Autodesk Fusion 360 part; units mm, degrees
note: some values were not read from the file. Chosen so that the rebuilt part matches the saved one: which bodies a step acts on.
(part 3 of 4)
sketch "BBB_22mm_Gearmotor_L_Section" plane through (0, 0, 0) normal (1, 0, 0) x (0, 0, -1) in component "BBB_22mm_Gearmotor_L"
  circle A0 centre (-21, 0) radius 11
extrude "Extrude1'''''''''''''''''''''''''''''''''''''''''''''''''''''''''''''''''''''" add sketch "BBB_22mm_Gearmotor_L_Section" along normal blind 49 from surface at -58 separate body makes body 78 in component "BBB_22mm_Gearmotor_L"
sketch "BBB_4mm_Output_Shaft_L_Section" plane through (0, 0, 0) normal (1, 0, 0) x (0, 0, -1) in component "BBB_4mm_Output_Shaft_L"
  circle A0 centre (-21, 0) radius 2
extrude "Extrude1''''''''''''''''''''''''''''''''''''''''''''''''''''''''''''''''''''''" add sketch "BBB_4mm_Output_Shaft_L_Section" along normal blind 14 from surface at -72 separate body makes body 79 in component "BBB_4mm_Output_Shaft_L"
sketch "BBB_Face_Mount_26mm_L_Outline" plane through (0, 0, 0) normal (0, 0, 1) x (1, 0, 0) in component "BBB_Face_Mount_26mm_L"
  line L0 (-61, -13) -> (-58, -13)
  line L1 (-58, -13) -> (-58, 13)
  line L2 (-58, 13) -> (-61, 13)
  line L3 (-61, 13) -> (-61, -13)
extrude "Extrude1'''''''''''''''''''''''''''''''''''''''''''''''''''''''''''''''''''''''" add sketch "BBB_Face_Mount_26mm_L_Outline" along normal blind 26 from surface at 8 separate body makes body 80 in component "BBB_Face_Mount_26mm_L"
sketch "Face_Motor_Bore_L" plane through (0, 0, 0) normal (1, 0, 0) x (0, 0, -1) in component "BBB_Face_Mount_26mm_L"
  circle A0 centre (-21, 0) radius 11.1
extrude "Face_Motor_Bore_L_Cut" cut sketch "Face_Motor_Bore_L" along normal blind 3.2 from surface at -61.1 bodies 80 in component "BBB_Face_Mount_26mm_L"
sketch "Face_M3_20mm_Pattern_L" plane through (0, 0, 0) normal (1, 0, 0) x (0, 0, -1) in component "BBB_Face_Mount_26mm_L"
  circle A0 centre (-11, -10) radius 1.6
  circle A1 centre (-31, -10) radius 1.6
  circle A2 centre (-11, 10) radius 1.6
  circle A3 centre (-31, 10) radius 1.6
extrude "Face_M3_20mm_Pattern_L_Cut" cut sketch "Face_M3_20mm_Pattern_L" along normal blind 3.2 from surface at -61.1 bodies 80 in component "BBB_Face_Mount_26mm_L"
sketch "BBB_Motor_Cradle_L_Outline" plane through (0, 0, 0) normal (0, 0, 1) x (1, 0, 0) in component "BBB_Motor_Cradle_L"
  line L0 (-58, -20) -> (-48, -20)
  line L1 (-48, -20) -> (-48, 20)
  line L2 (-48, 20) -> (-58, 20)
  line L3 (-58, 20) -> (-58, -20)
extrude "Extrude1''''''''''''''''''''''''''''''''''''''''''''''''''''''''''''''''''''''''" add sketch "BBB_Motor_Cradle_L_Outline" along normal blind 32 from surface at 5 separate body makes body 81 in component "BBB_Motor_Cradle_L"
sketch "Cradle_Motor_Bore_L" plane through (0, 0, 0) normal (1, 0, 0) x (0, 0, -1) in component "BBB_Motor_Cradle_L"
  circle A0 centre (-21, 0) radius 11.1
extrude "Cradle_Motor_Bore_L_Cut" cut sketch "Cradle_Motor_Bore_L" along normal blind 10.2 from surface at -58.1 bodies 81 in component "BBB_Motor_Cradle_L"
sketch "Cradle_M3_Face_Tap_L" plane through (0, 0, 0) normal (1, 0, 0) x (0, 0, -1) in component "BBB_Motor_Cradle_L"
  circle A0 centre (-11, -10) radius 1.25
  circle A1 centre (-31, -10) radius 1.25
  circle A2 centre (-11, 10) radius 1.25
  circle A3 centre (-31, 10) radius 1.25
extrude "Cradle_M3_Face_Tap_L_Cut" cut sketch "Cradle_M3_Face_Tap_L" along normal blind 10.2 from surface at -58.1 bodies 81 in component "BBB_Motor_Cradle_L"
sketch "Cradle_M3_Base_Tap_L" plane through (0, 0, 0) normal (0, 0, 1) x (1, 0, 0) in component "BBB_Motor_Cradle_L"
  circle A0 centre (-53, -16) radius 1.25
  circle A1 centre (-53, 16) radius 1.25
extrude "Cradle_M3_Base_Tap_L_Cut" cut sketch "Cradle_M3_Base_Tap_L" along normal blind 12.1 from surface at 4.9 bodies 81 in component "BBB_Motor_Cradle_L"
sketch "Cradle_M3_Base_Clear_L" plane through (0, 0, 0) normal (0, 0, 1) x (1, 0, 0) in component "Base_Plate_Al"
  circle A0 centre (-53, -16) radius 1.7
  circle A1 centre (-53, 16) radius 1.7
extrude "Cradle_M3_Base_Clear_L_Cut" cut sketch "Cradle_M3_Base_Clear_L" along normal blind 2.2 from surface at 2.9 bodies 1 in component "Base_Plate_Al"
sketch "Hub_16p2_Counterbore_L" plane through (0, 0, 0) normal (1, 0, 0) x (0, 0, -1) in component "Left_Wheel"
  circle A0 centre (-21, 0) radius 8.1
extrude "Hub_16p2_Counterbore_L_Cut" cut sketch "Hub_16p2_Counterbore_L" along normal blind 6.4 from surface at -67.2 bodies 4 in component "Left_Wheel"
sketch "Shaft_4p2_Blind_Bore_L" plane through (0, 0, 0) normal (1, 0, 0) x (0, 0, -1) in component "Left_Wheel"
  circle A0 centre (-21, 0) radius 2.1
extrude "Shaft_4p2_Blind_Bore_L_Cut" cut sketch "Shaft_4p2_Blind_Bore_L" along normal blind 5.1 from surface at -72.2 bodies 4 in component "Left_Wheel"
sketch "Wheel_M3_12p7_Pattern_L" plane through (0, 0, 0) normal (1, 0, 0) x (0, 0, -1) in component "Left_Wheel"
  circle A0 centre (-21, -6.35) radius 1.7
  circle A1 centre (-21, 6.35) radius 1.7
extrude "Wheel_M3_12p7_Pattern_L_Cut" cut sketch "Wheel_M3_12p7_Pattern_L" along normal blind 13 from surface at -80.1 bodies 4 in component "Left_Wheel"
sketch "Repeat_4mm_Clamp_Hub_L_Section" plane through (0, 0, 0) normal (1, 0, 0) x (0, 0, -1) in component "Repeat_4mm_Clamp_Hub_L"
  circle A0 centre (-21, 0) radius 8
extrude "Extrude1'''''''''''''''''''''''''''''''''''''''''''''''''''''''''''''''''''''''''" add sketch "Repeat_4mm_Clamp_Hub_L_Section" along normal blind 6 from surface at -67 separate body makes body 82 in component "Repeat_4mm_Clamp_Hub_L"
sketch "Hub_4mm_Shaft_Bore_L" plane through (0, 0, 0) normal (1, 0, 0) x (0, 0, -1) in component "Repeat_4mm_Clamp_Hub_L"
  circle A0 centre (-21, 0) radius 2
extrude "Hub_4mm_Shaft_Bore_L_Cut" cut sketch "Hub_4mm_Shaft_Bore_L" along normal blind 6.2 from surface at -67.1 bodies 82 in component "Repeat_4mm_Clamp_Hub_L"
sketch "Hub_M3_12p7_Tap_L" plane through (0, 0, 0) normal (1, 0, 0) x (0, 0, -1) in component "Repeat_4mm_Clamp_Hub_L"
  circle A0 centre (-21, -6.35) radius 1.25
  circle A1 centre (-21, 6.35) radius 1.25
extrude "Hub_M3_12p7_Tap_L_Cut" cut sketch "Hub_M3_12p7_Tap_L" along normal blind 6.2 from surface at -67.1 bodies 82 in component "Repeat_4mm_Clamp_Hub_L"
sketch "BBB_22mm_Gearmotor_R_Section" plane through (0, 0, 0) normal (1, 0, 0) x (0, 0, -1) in component "BBB_22mm_Gearmotor_R"
  circle A0 centre (-21, 0) radius 11
extrude "Extrude1''''''''''''''''''''''''''''''''''''''''''''''''''''''''''''''''''''''''''" add sketch "BBB_22mm_Gearmotor_R_Section" along normal blind 49 from surface at 9 separate body makes body 83 in component "BBB_22mm_Gearmotor_R"
sketch "BBB_4mm_Output_Shaft_R_Section" plane through (0, 0, 0) normal (1, 0, 0) x (0, 0, -1) in component "BBB_4mm_Output_Shaft_R"
  circle A0 centre (-21, 0) radius 2
extrude "Extrude1'''''''''''''''''''''''''''''''''''''''''''''''''''''''''''''''''''''''''''" add sketch "BBB_4mm_Output_Shaft_R_Section" along normal blind 14 from surface at 58 separate body makes body 84 in component "BBB_4mm_Output_Shaft_R"
sketch "BBB_Face_Mount_26mm_R_Outline" plane through (0, 0, 0) normal (0, 0, 1) x (1, 0, 0) in component "BBB_Face_Mount_26mm_R"
  line L0 (58, -13) -> (61, -13)
  line L1 (61, -13) -> (61, 13)
  line L2 (61, 13) -> (58, 13)
  line L3 (58, 13) -> (58, -13)
extrude "Extrude1''''''''''''''''''''''''''''''''''''''''''''''''''''''''''''''''''''''''''''" add sketch "BBB_Face_Mount_26mm_R_Outline" along normal blind 26 from surface at 8 separate body makes body 85 in component "BBB_Face_Mount_26mm_R"
sketch "Face_Motor_Bore_R" plane through (0, 0, 0) normal (1, 0, 0) x (0, 0, -1) in component "BBB_Face_Mount_26mm_R"
  circle A0 centre (-21, 0) radius 11.1
extrude "Face_Motor_Bore_R_Cut" cut sketch "Face_Motor_Bore_R" along normal blind 3.2 from surface at 57.9 bodies 85 in component "BBB_Face_Mount_26mm_R"
sketch "Face_M3_20mm_Pattern_R" plane through (0, 0, 0) normal (1, 0, 0) x (0, 0, -1) in component "BBB_Face_Mount_26mm_R"
  circle A0 centre (-11, -10) radius 1.6
  circle A1 centre (-31, -10) radius 1.6
  circle A2 centre (-11, 10) radius 1.6
  circle A3 centre (-31, 10) radius 1.6
extrude "Face_M3_20mm_Pattern_R_Cut" cut sketch "Face_M3_20mm_Pattern_R" along normal blind 3.2 from surface at 57.9 bodies 85 in component "BBB_Face_Mount_26mm_R"
sketch "BBB_Motor_Cradle_R_Outline" plane through (0, 0, 0) normal (0, 0, 1) x (1, 0, 0) in component "BBB_Motor_Cradle_R"
  line L0 (48, -20) -> (58, -20)
  line L1 (58, -20) -> (58, 20)
  line L2 (58, 20) -> (48, 20)
  line L3 (48, 20) -> (48, -20)
extrude "Extrude1'''''''''''''''''''''''''''''''''''''''''''''''''''''''''''''''''''''''''''''" add sketch "BBB_Motor_Cradle_R_Outline" along normal blind 32 from surface at 5 separate body makes body 86 in component "BBB_Motor_Cradle_R"
sketch "Cradle_Motor_Bore_R" plane through (0, 0, 0) normal (1, 0, 0) x (0, 0, -1) in component "BBB_Motor_Cradle_R"
  circle A0 centre (-21, 0) radius 11.1
extrude "Cradle_Motor_Bore_R_Cut" cut sketch "Cradle_Motor_Bore_R" along normal blind 10.2 from surface at 47.9 bodies 86 in component "BBB_Motor_Cradle_R"
sketch "Cradle_M3_Face_Tap_R" plane through (0, 0, 0) normal (1, 0, 0) x (0, 0, -1) in component "BBB_Motor_Cradle_R"
  circle A0 centre (-11, -10) radius 1.25
  circle A1 centre (-31, -10) radius 1.25
  circle A2 centre (-11, 10) radius 1.25
  circle A3 centre (-31, 10) radius 1.25
extrude "Cradle_M3_Face_Tap_R_Cut" cut sketch "Cradle_M3_Face_Tap_R" along normal blind 10.2 from surface at 47.9 bodies 86 in component "BBB_Motor_Cradle_R"
sketch "Cradle_M3_Base_Tap_R" plane through (0, 0, 0) normal (0, 0, 1) x (1, 0, 0) in component "BBB_Motor_Cradle_R"
  circle A0 centre (53, -16) radius 1.25
  circle A1 centre (53, 16) radius 1.25
extrude "Cradle_M3_Base_Tap_R_Cut" cut sketch "Cradle_M3_Base_Tap_R" along normal blind 12.1 from surface at 4.9 bodies 86 in component "BBB_Motor_Cradle_R"
sketch "Cradle_M3_Base_Clear_R" plane through (0, 0, 0) normal (0, 0, 1) x (1, 0, 0) in component "Base_Plate_Al"
  circle A0 centre (53, -16) radius 1.7
  circle A1 centre (53, 16) radius 1.7
extrude "Cradle_M3_Base_Clear_R_Cut" cut sketch "Cradle_M3_Base_Clear_R" along normal blind 2.2 from surface at 2.9 bodies 1 in component "Base_Plate_Al"
sketch "Hub_16p2_Counterbore_R" plane through (0, 0, 0) normal (1, 0, 0) x (0, 0, -1) in component "Right_Wheel"
  circle A0 centre (-21, 0) radius 8.1
extrude "Hub_16p2_Counterbore_R_Cut" cut sketch "Hub_16p2_Counterbore_R" along normal blind 6.4 from surface at 60.8 bodies 5 in component "Right_Wheel"
sketch "Shaft_4p2_Blind_Bore_R" plane through (0, 0, 0) normal (1, 0, 0) x (0, 0, -1) in component "Right_Wheel"
  circle A0 centre (-21, 0) radius 2.1
extrude "Shaft_4p2_Blind_Bore_R_Cut" cut sketch "Shaft_4p2_Blind_Bore_R" along normal blind 5.1 from surface at 67.1 bodies 5 in component "Right_Wheel"
sketch "Wheel_M3_12p7_Pattern_R" plane through (0, 0, 0) normal (1, 0, 0) x (0, 0, -1) in component "Right_Wheel"
  circle A0 centre (-21, -6.35) radius 1.7
  circle A1 centre (-21, 6.35) radius 1.7
extrude "Wheel_M3_12p7_Pattern_R_Cut" cut sketch "Wheel_M3_12p7_Pattern_R" along normal blind 13 from surface at 67.1 bodies 5 in component "Right_Wheel"
sketch "Repeat_4mm_Clamp_Hub_R_Section" plane through (0, 0, 0) normal (1, 0, 0) x (0, 0, -1) in component "Repeat_4mm_Clamp_Hub_R"
  circle A0 centre (-21, 0) radius 8
extrude "Extrude1''''''''''''''''''''''''''''''''''''''''''''''''''''''''''''''''''''''''''''''" add sketch "Repeat_4mm_Clamp_Hub_R_Section" along normal blind 6 from surface at 61 separate body makes body 87 in component "Repeat_4mm_Clamp_Hub_R"
sketch "Hub_4mm_Shaft_Bore_R" plane through (0, 0, 0) normal (1, 0, 0) x (0, 0, -1) in component "Repeat_4mm_Clamp_Hub_R"
  circle A0 centre (-21, 0) radius 2
extrude "Hub_4mm_Shaft_Bore_R_Cut" cut sketch "Hub_4mm_Shaft_Bore_R" along normal blind 6.2 from surface at 60.9 bodies 87 in component "Repeat_4mm_Clamp_Hub_R"
sketch "Hub_M3_12p7_Tap_R" plane through (0, 0, 0) normal (1, 0, 0) x (0, 0, -1) in component "Repeat_4mm_Clamp_Hub_R"
  circle A0 centre (-21, -6.35) radius 1.25
  circle A1 centre (-21, 6.35) radius 1.25
extrude "Hub_M3_12p7_Tap_R_Cut" cut sketch "Hub_M3_12p7_Tap_R" along normal blind 6.2 from surface at 60.9 bodies 87 in component "Repeat_4mm_Clamp_Hub_R"
sketch "BBB_Dual_Brushed_ESC_v2_Envelope_Outline" plane through (0, 0, 0) normal (0, 0, 1) x (1, 0, 0) in component "BBB_Dual_Brushed_ESC_v2_Envelope"
  line L0 (-8, -84) -> (12, -84)
  line L1 (12, -84) -> (12, -68)
  line L2 (12, -68) -> (-8, -68)
  line L3 (-8, -68) -> (-8, -84)
extrude "Extrude1'''''''''''''''''''''''''''''''''''''''''''''''''''''''''''''''''''''''''''''''" add sketch "BBB_Dual_Brushed_ESC_v2_Envelope_Outline" along normal blind 5 from surface at 7 separate body makes body 88 in component "BBB_Dual_Brushed_ESC_v2_Envelope"
sketch "Battery_Tray_Rear_Clearance_L" plane through (0, 0, 0) normal (0, 0, 1) x (1, 0, 0) in component "BBB_Motor_Cradle_L"
  line L0 (-58.1, -20.1) -> (-47.9, -20.1)
  line L1 (-47.9, -20.1) -> (-47.9, -18)
  line L2 (-47.9, -18) -> (-58.1, -18)
  line L3 (-58.1, -18) -> (-58.1, -20.1)
extrude "Extrude5''''''''''''''" cut sketch "Battery_Tray_Rear_Clearance_L" along normal blind 7.1 from surface at 30 bodies 81 in component "BBB_Motor_Cradle_L"
sketch "Battery_Tray_Rear_Clearance_R" plane through (0, 0, 0) normal (0, 0, 1) x (1, 0, 0) in component "BBB_Motor_Cradle_R"
  line L0 (47.9, -20.1) -> (58.1, -20.1)
  line L1 (58.1, -20.1) -> (58.1, -18)
  line L2 (58.1, -18) -> (47.9, -18)
  line L3 (47.9, -18) -> (47.9, -20.1)
extrude "Extrude5'''''''''''''''" cut sketch "Battery_Tray_Rear_Clearance_R" along normal blind 7.1 from surface at 30 bodies 86 in component "BBB_Motor_Cradle_R"
sketch "Battery_Clamp_Bar_1_Outline" plane through (0, 0, 0) normal (0, 0, 1) x (1, 0, 0) in component "Battery_Clamp_Bar_1"
  line L0 (-78, -51) -> (78, -51)
  line L1 (78, -51) -> (78, -45)
  line L2 (78, -45) -> (-78, -45)
  line L3 (-78, -45) -> (-78, -51)
extrude "Extrude1''''''''''''''''''''''''''''''''''''''''''''''''''''''''''''''''''''''''''''''''" add sketch "Battery_Clamp_Bar_1_Outline" along normal blind 6 from surface at 61.6 separate body makes body 89 in component "Battery_Clamp_Bar_1"
sketch "Clamp_M3_Tap_L_1" plane through (0, 0, 0) normal (1, 0, 0) x (0, 0, -1) in component "Battery_Clamp_Bar_1"
  circle A0 centre (-64.6, -48) radius 1.25
extrude "Extrude2'''''''''''''''''''''''''''''''''''''''''''''''''" cut sketch "Clamp_M3_Tap_L_1" along normal blind 10.2 from surface at -78.1 bodies 89 in component "Battery_Clamp_Bar_1"
sketch "Clamp_M3_Tap_R_1" plane through (0, 0, 0) normal (1, 0, 0) x (0, 0, -1) in component "Battery_Clamp_Bar_1"
  circle A0 centre (-64.6, -48) radius 1.25
extrude "Extrude3''''''''''''''''''''''''''''" cut sketch "Clamp_M3_Tap_R_1" along normal blind 10.2 from surface at 67.9 bodies 89 in component "Battery_Clamp_Bar_1"
sketch "Clamp_M3_Clear_L_1" plane through (0, 0, 0) normal (1, 0, 0) x (0, 0, -1) in component "Left_Side_Plate_Al"
  circle A0 centre (-64.6, -48) radius 1.7
extrude "Extrude8'''" cut sketch "Clamp_M3_Clear_L_1" along normal blind 2.2 from surface at -80.1 bodies 2 in component "Left_Side_Plate_Al"
sketch "Clamp_M3_Clear_R_1" plane through (0, 0, 0) normal (1, 0, 0) x (0, 0, -1) in component "Right_Side_Plate_Al"
  circle A0 centre (-64.6, -48) radius 1.7
extrude "Extrude8''''" cut sketch "Clamp_M3_Clear_R_1" along normal blind 2.2 from surface at 77.9 bodies 3 in component "Right_Side_Plate_Al"
sketch "Battery_Clamp_Bar_2_Outline" plane through (0, 0, 0) normal (0, 0, 1) x (1, 0, 0) in component "Battery_Clamp_Bar_2"
  line L0 (-78, -31) -> (78, -31)
  line L1 (78, -31) -> (78, -25)
  line L2 (78, -25) -> (-78, -25)
  line L3 (-78, -25) -> (-78, -31)
extrude "Extrude1'''''''''''''''''''''''''''''''''''''''''''''''''''''''''''''''''''''''''''''''''" add sketch "Battery_Clamp_Bar_2_Outline" along normal blind 6 from surface at 61.6 separate body makes body 90 in component "Battery_Clamp_Bar_2"
sketch "Clamp_M3_Tap_L_2" plane through (0, 0, 0) normal (1, 0, 0) x (0, 0, -1) in component "Battery_Clamp_Bar_2"
  circle A0 centre (-64.6, -28) radius 1.25
extrude "Extrude2''''''''''''''''''''''''''''''''''''''''''''''''''" cut sketch "Clamp_M3_Tap_L_2" along normal blind 10.2 from surface at -78.1 bodies 90 in component "Battery_Clamp_Bar_2"
sketch "Clamp_M3_Tap_R_2" plane through (0, 0, 0) normal (1, 0, 0) x (0, 0, -1) in component "Battery_Clamp_Bar_2"
  circle A0 centre (-64.6, -28) radius 1.25
extrude "Extrude3'''''''''''''''''''''''''''''" cut sketch "Clamp_M3_Tap_R_2" along normal blind 10.2 from surface at 67.9 bodies 90 in component "Battery_Clamp_Bar_2"
sketch "Clamp_M3_Clear_L_2" plane through (0, 0, 0) normal (1, 0, 0) x (0, 0, -1) in component "Left_Side_Plate_Al"
  circle A0 centre (-64.6, -28) radius 1.7
extrude "Extrude9'" cut sketch "Clamp_M3_Clear_L_2" along normal blind 2.2 from surface at -80.1 bodies 2 in component "Left_Side_Plate_Al"
sketch "Clamp_M3_Clear_R_2" plane through (0, 0, 0) normal (1, 0, 0) x (0, 0, -1) in component "Right_Side_Plate_Al"
  circle A0 centre (-64.6, -28) radius 1.7
extrude "Extrude9''" cut sketch "Clamp_M3_Clear_R_2" along normal blind 2.2 from surface at 77.9 bodies 3 in component "Right_Side_Plate_Al"
sketch "Lifter_Servo_Clamp_Bar_L_Outline" plane through (0, 0, 0) normal (0, 0, 1) x (1, 0, 0) in component "Lifter_Servo_Clamp_Bar_L"
  line L0 (-15, -15) -> (-9, -15)
  line L1 (-9, -15) -> (-9, 60)
  line L2 (-9, 60) -> (-15, 60)
  line L3 (-15, 60) -> (-15, -15)
extrude "Extrude1''''''''''''''''''''''''''''''''''''''''''''''''''''''''''''''''''''''''''''''''''" add sketch "Lifter_Servo_Clamp_Bar_L_Outline" along normal blind 2 from surface at 32 separate body makes body 91 in component "Lifter_Servo_Clamp_Bar_L"
sketch "Clamp_Bar_M3_Clear_L" plane through (0, 0, 0) normal (0, 0, 1) x (1, 0, 0) in component "Lifter_Servo_Clamp_Bar_L"
  circle A0 centre (-12, -15) radius 1.7
  circle A1 centre (-12, 60) radius 1.7
extrude "Extrude2'''''''''''''''''''''''''''''''''''''''''''''''''''" cut sketch "Clamp_Bar_M3_Clear_L" along normal blind 2.2 from surface at 31.9 bodies 91 in component "Lifter_Servo_Clamp_Bar_L"
sketch "Lifter_Servo_Clamp_Post_L_Rear_Outline" plane through (0, 0, 0) normal (0, 0, 1) x (1, 0, 0) in component "Lifter_Servo_Clamp_Post_L_Rear"
  line L0 (-15, -18) -> (-9, -18)
  line L1 (-9, -18) -> (-9, -12)
  line L2 (-9, -12) -> (-15, -12)
  line L3 (-15, -12) -> (-15, -18)
extrude "Extrude1'''''''''''''''''''''''''''''''''''''''''''''''''''''''''''''''''''''''''''''''''''" add sketch "Lifter_Servo_Clamp_Post_L_Rear_Outline" along normal blind 27 from surface at 5 separate body makes body 92 in component "Lifter_Servo_Clamp_Post_L_Rear"
sketch "Clamp_Post_M3_Tap_L_Rear" plane through (0, 0, 0) normal (0, 0, 1) x (1, 0, 0) in component "Lifter_Servo_Clamp_Post_L_Rear"
  circle A0 centre (-12, -15) radius 1.25
extrude "Extrude2''''''''''''''''''''''''''''''''''''''''''''''''''''" cut sketch "Clamp_Post_M3_Tap_L_Rear" along normal blind 27.2 from surface at 4.9 bodies 92 in component "Lifter_Servo_Clamp_Post_L_Rear"
sketch "Lifter_Servo_Clamp_Post_L_Front_Outline" plane through (0, 0, 0) normal (0, 0, 1) x (1, 0, 0) in component "Lifter_Servo_Clamp_Post_L_Front"
  line L0 (-15, 57) -> (-9, 57)
  line L1 (-9, 57) -> (-9, 63)
  line L2 (-9, 63) -> (-15, 63)
  line L3 (-15, 63) -> (-15, 57)
extrude "Extrude1''''''''''''''''''''''''''''''''''''''''''''''''''''''''''''''''''''''''''''''''''''" add sketch "Lifter_Servo_Clamp_Post_L_Front_Outline" along normal blind 27 from surface at 5 separate body makes body 93 in component "Lifter_Servo_Clamp_Post_L_Front"
sketch "Clamp_Post_M3_Tap_L_Front" plane through (0, 0, 0) normal (0, 0, 1) x (1, 0, 0) in component "Lifter_Servo_Clamp_Post_L_Front"
  circle A0 centre (-12, 60) radius 1.25
extrude "Extrude2'''''''''''''''''''''''''''''''''''''''''''''''''''''" cut sketch "Clamp_Post_M3_Tap_L_Front" along normal blind 27.2 from surface at 4.9 bodies 93 in component "Lifter_Servo_Clamp_Post_L_Front"
sketch "Lifter_Servo_Clamp_Bar_R_Outline" plane through (0, 0, 0) normal (0, 0, 1) x (1, 0, 0) in component "Lifter_Servo_Clamp_Bar_R"
  line L0 (9, -15) -> (15, -15)
  line L1 (15, -15) -> (15, 60)
  line L2 (15, 60) -> (9, 60)
  line L3 (9, 60) -> (9, -15)
extrude "Extrude1'''''''''''''''''''''''''''''''''''''''''''''''''''''''''''''''''''''''''''''''''''''" add sketch "Lifter_Servo_Clamp_Bar_R_Outline" along normal blind 2 from surface at 32 separate body makes body 94 in component "Lifter_Servo_Clamp_Bar_R"
sketch "Clamp_Bar_M3_Clear_R" plane through (0, 0, 0) normal (0, 0, 1) x (1, 0, 0) in component "Lifter_Servo_Clamp_Bar_R"
  circle A0 centre (12, -15) radius 1.7
  circle A1 centre (12, 60) radius 1.7
extrude "Extrude2''''''''''''''''''''''''''''''''''''''''''''''''''''''" cut sketch "Clamp_Bar_M3_Clear_R" along normal blind 2.2 from surface at 31.9 bodies 94 in component "Lifter_Servo_Clamp_Bar_R"
sketch "Lifter_Servo_Clamp_Post_R_Rear_Outline" plane through (0, 0, 0) normal (0, 0, 1) x (1, 0, 0) in component "Lifter_Servo_Clamp_Post_R_Rear"
  line L0 (9, -18) -> (15, -18)
  line L1 (15, -18) -> (15, -12)
  line L2 (15, -12) -> (9, -12)
  line L3 (9, -12) -> (9, -18)
extrude "Extrude1''''''''''''''''''''''''''''''''''''''''''''''''''''''''''''''''''''''''''''''''''''''" add sketch "Lifter_Servo_Clamp_Post_R_Rear_Outline" along normal blind 27 from surface at 5 separate body makes body 95 in component "Lifter_Servo_Clamp_Post_R_Rear"
sketch "Clamp_Post_M3_Tap_R_Rear" plane through (0, 0, 0) normal (0, 0, 1) x (1, 0, 0) in component "Lifter_Servo_Clamp_Post_R_Rear"
  circle A0 centre (12, -15) radius 1.25
extrude "Extrude2'''''''''''''''''''''''''''''''''''''''''''''''''''''''" cut sketch "Clamp_Post_M3_Tap_R_Rear" along normal blind 27.2 from surface at 4.9 bodies 95 in component "Lifter_Servo_Clamp_Post_R_Rear"
sketch "Lifter_Servo_Clamp_Post_R_Front_Outline" plane through (0, 0, 0) normal (0, 0, 1) x (1, 0, 0) in component "Lifter_Servo_Clamp_Post_R_Front"
  line L0 (9, 57) -> (15, 57)
  line L1 (15, 57) -> (15, 63)
  line L2 (15, 63) -> (9, 63)
  line L3 (9, 63) -> (9, 57)
extrude "Extrude1'''''''''''''''''''''''''''''''''''''''''''''''''''''''''''''''''''''''''''''''''''''''" add sketch "Lifter_Servo_Clamp_Post_R_Front_Outline" along normal blind 27 from surface at 5 separate body makes body 96 in component "Lifter_Servo_Clamp_Post_R_Front"
sketch "Clamp_Post_M3_Tap_R_Front" plane through (0, 0, 0) normal (0, 0, 1) x (1, 0, 0) in component "Lifter_Servo_Clamp_Post_R_Front"
  circle A0 centre (12, 60) radius 1.25
extrude "Extrude2''''''''''''''''''''''''''''''''''''''''''''''''''''''''" cut sketch "Clamp_Post_M3_Tap_R_Front" along normal blind 27.2 from surface at 4.9 bodies 96 in component "Lifter_Servo_Clamp_Post_R_Front"
sketch "Lifter_Servo_Clamp_Base_M3_Clear" plane through (0, 0, 0) normal (0, 0, 1) x (1, 0, 0) in component "Base_Plate_Al"
  circle A0 centre (-12, -15) radius 1.7
  circle A1 centre (-12, 60) radius 1.7
  circle A2 centre (12, -15) radius 1.7
  circle A3 centre (12, 60) radius 1.7
extrude "Extrude33" cut sketch "Lifter_Servo_Clamp_Base_M3_Clear" along normal blind 2.2 from surface at 2.9 bodies 1 in component "Base_Plate_Al"
sketch "Pin_Clip_Groove_L" plane through (0, 0, 0) normal (1, 0, 0) x (0, 0, -1) in component "Lifter_Pivot_Pin_6mm"
  circle A0 centre (-31.5, 68) radius 3.05
  circle A1 centre (-31.5, 68) radius 2.5
extrude "Extrude4''''''''''''''''''''" cut sketch "Pin_Clip_Groove_L" along normal blind 0.8 from surface at -31.4 bodies 60 in component "Lifter_Pivot_Pin_6mm"
sketch "Pin_Clip_Groove_R" plane through (0, 0, 0) normal (1, 0, 0) x (0, 0, -1) in component "Lifter_Pivot_Pin_6mm"
  circle A0 centre (-31.5, 68) radius 3.05
  circle A1 centre (-31.5, 68) radius 2.5
extrude "Extrude5''''''''''''''''" cut sketch "Pin_Clip_Groove_R" along normal blind 0.8 from surface at 30.6 bodies 60 in component "Lifter_Pivot_Pin_6mm"
sketch "C_Clip_Section_L" plane through (0, 0, 0) normal (1, 0, 0) x (0, 0, -1) in component "Lifter_Pin_C_Clip_L"
  circle A0 centre (-31.5, 68) radius 5
  circle A1 centre (-31.5, 68) radius 2.5
extrude "Extrude1''''''''''''''''''''''''''''''''''''''''''''''''''''''''''''''''''''''''''''''''''''''''" add sketch "C_Clip_Section_L" along normal blind 0.8 from surface at -31.4 separate body makes body 97 in component "Lifter_Pin_C_Clip_L"
sketch "C_Clip_Opening_L" plane through (0, 0, 0) normal (1, 0, 0) x (0, 0, -1) in component "Lifter_Pin_C_Clip_L"
  line L0 (-30.4, 70.2) -> (-32.6, 70.2)
  line L1 (-32.6, 70.2) -> (-32.6, 73.2)
  line L2 (-32.6, 73.2) -> (-30.4, 73.2)
  line L3 (-30.4, 73.2) -> (-30.4, 70.2)
extrude "Extrude2'''''''''''''''''''''''''''''''''''''''''''''''''''''''''" cut sketch "C_Clip_Opening_L" along normal blind 1 from surface at -31.5 bodies 97 in component "Lifter_Pin_C_Clip_L"
sketch "C_Clip_Section_R" plane through (0, 0, 0) normal (1, 0, 0) x (0, 0, -1) in component "Lifter_Pin_C_Clip_R"
  circle A0 centre (-31.5, 68) radius 5
  circle A1 centre (-31.5, 68) radius 2.5
extrude "Extrude1'''''''''''''''''''''''''''''''''''''''''''''''''''''''''''''''''''''''''''''''''''''''''" add sketch "C_Clip_Section_R" along normal blind 0.8 from surface at 30.6 separate body makes body 98 in component "Lifter_Pin_C_Clip_R"
sketch "C_Clip_Opening_R" plane through (0, 0, 0) normal (1, 0, 0) x (0, 0, -1) in component "Lifter_Pin_C_Clip_R"
  line L0 (-30.4, 70.2) -> (-32.6, 70.2)
  line L1 (-32.6, 70.2) -> (-32.6, 73.2)
  line L2 (-32.6, 73.2) -> (-30.4, 73.2)
  line L3 (-30.4, 73.2) -> (-30.4, 70.2)
extrude "Extrude2''''''''''''''''''''''''''''''''''''''''''''''''''''''''''" cut sketch "C_Clip_Opening_R" along normal blind 1 from surface at 30.5 bodies 98 in component "Lifter_Pin_C_Clip_R"
sketch "C_Clip_OD_8p4_L" plane through (0, 0, 0) normal (1, 0, 0) x (0, 0, -1) in component "Lifter_Pin_C_Clip_L"
  circle A0 centre (-31.5, 68) radius 5.1
  circle A1 centre (-31.5, 68) radius 4.2
extrude "Extrude3''''''''''''''''''''''''''''''" cut sketch "C_Clip_OD_8p4_L" along normal blind 1 from surface at -31.5 bodies 97 in component "Lifter_Pin_C_Clip_L"
sketch "C_Clip_OD_8p4_R" plane through (0, 0, 0) normal (1, 0, 0) x (0, 0, -1) in component "Lifter_Pin_C_Clip_R"
  circle A0 centre (-31.5, 68) radius 5.1
  circle A1 centre (-31.5, 68) radius 4.2
extrude "Extrude3'''''''''''''''''''''''''''''''" cut sketch "C_Clip_OD_8p4_R" along normal blind 1 from surface at 30.5 bodies 98 in component "Lifter_Pin_C_Clip_R"
sketch "C_Clip_OD_8p0_L" plane through (0, 0, 0) normal (1, 0, 0) x (0, 0, -1) in component "Lifter_Pin_C_Clip_L"
  circle A0 centre (-31.5, 68) radius 5.1
  circle A1 centre (-31.5, 68) radius 4
extrude "Extrude4'''''''''''''''''''''" cut sketch "C_Clip_OD_8p0_L" along normal blind 1 from surface at -31.5 bodies 97 in component "Lifter_Pin_C_Clip_L"
sketch "C_Clip_OD_8p0_R" plane through (0, 0, 0) normal (1, 0, 0) x (0, 0, -1) in component "Lifter_Pin_C_Clip_R"
  circle A0 centre (-31.5, 68) radius 5.1
  circle A1 centre (-31.5, 68) radius 4
extrude "Extrude4''''''''''''''''''''''" cut sketch "C_Clip_OD_8p0_R" along normal blind 1 from surface at 30.5 bodies 98 in component "Lifter_Pin_C_Clip_R"
component "01_Chassis" placed x (1, 0, 0) y (0, 1, 0) z (0, 0, 1) at (0, 0, 0)
component "02_Drivetrain" placed x (1, 0, 0) y (0, 1, 0) z (0, 0, 1) at (0, 0, 0)
component "03_Front_Spinner" placed x (1, 0, 0) y (0, 1, 0) z (0, 0, 1) at (0, 0, 0)
component "05_Electronics" placed x (1, 0, 0) y (0, 1, 0) z (0, 0, 1) at (0, 0, 0)
component "06_3D_Printed" placed x (1, 0, 0) y (0, 1, 0) z (0, 0, 1) at (0, 0, 0)
component "07_Wedge_Lifter_Option" placed x (1, 0, 0) y (0, 1, 0) z (0, 0, 1) at (0, 0, 0)
component "08_Grabber_Addon_Option" placed x (1, 0, 0) y (0, 1, 0) z (0, 0, 1) at (0, 0, 0)
component "09_3S_Drive_Upgrade" placed x (1, 0, 0) y (0, 1, 0) z (0, 0, 1) at (0, 0, 0)
component "10_Battery_Restraints" placed x (1, 0, 0) y (0, 1, 0) z (0, 0, 1) at (0, 0, 0)
component "Base_Plate_Al" placed x (1, 0, 0) y (0, 1, 0) z (0, 0, 1) at (0, 0, 0) in component "01_Chassis"
component "Left_Side_Plate_Al" placed x (1, 0, 0) y (0, 1, 0) z (0, 0, 1) at (0, 0, 0) in component "01_Chassis"
component "Right_Side_Plate_Al" placed x (1, 0, 0) y (0, 1, 0) z (0, 0, 1) at (0, 0, 0) in component "01_Chassis"
component "Top_Cover" placed x (1, 0, 0) y (0, 1, 0) z (0, 0, 1) at (0, 0, 0) in component "01_Chassis"
component "Front_Wedge_L" placed x (1, 0, 0) y (0, 1, 0) z (0, 0, 1) at (0, 0, 0) in component "01_Chassis"
component "Front_Wedge_R" placed x (1, 0, 0) y (0, 1, 0) z (0, 0, 1) at (0, 0, 0) in component "01_Chassis"
component "Standoffs_Fasteners" placed x (1, 0, 0) y (0, 1, 0) z (0, 0, 1) at (0, 0, 0) in component "01_Chassis"
component "Left_Wheel" placed x (1, 0, 0) y (0, 1, 0) z (0, 0, 1) at (0, 0, 0) in component "02_Drivetrain"
component "Right_Wheel" placed x (1, 0, 0) y (0, 1, 0) z (0, 0, 1) at (0, 0, 0) in component "02_Drivetrain"
component "TT_Gearbox_L" placed x (1, 0, 0) y (0, 1, 0) z (0, 0, 1) at (0, 0, 0) in component "02_Drivetrain"
component "TT_Motor_Can_L" placed x (1, 0, 0) y (0, 1, 0) z (0, 0, 1) at (0, 0, 0) in component "02_Drivetrain"
component "TT_Gearbox_R" placed x (1, 0, 0) y (0, 1, 0) z (0, 0, 1) at (0, 0, 0) in component "02_Drivetrain"
component "TT_Motor_Can_R" placed x (1, 0, 0) y (0, 1, 0) z (0, 0, 1) at (0, 0, 0) in component "02_Drivetrain"
component "TT_Motor_Mount_L" placed x (1, 0, 0) y (0, 1, 0) z (0, 0, 1) at (0, 0, 0) in component "02_Drivetrain"
component "TT_Motor_Clamp_L" placed x (1, 0, 0) y (0, 1, 0) z (0, 0, 1) at (0, 0, 0) in component "02_Drivetrain"
component "TT_Motor_Mount_R" placed x (1, 0, 0) y (0, 1, 0) z (0, 0, 1) at (0, 0, 0) in component "02_Drivetrain"
component "TT_Motor_Clamp_R" placed x (1, 0, 0) y (0, 1, 0) z (0, 0, 1) at (0, 0, 0) in component "02_Drivetrain"
component "Spinner_Shaft" placed x (1, 0, 0) y (0, 1, 0) z (0, 0, 1) at (0, 0, 0) in component "03_Front_Spinner"
component "Left_Support" placed x (1, 0, 0) y (0, 1, 0) z (0, 0, 1) at (0, 0, 0) in component "03_Front_Spinner"
component "Right_Support" placed x (1, 0, 0) y (0, 1, 0) z (0, 0, 1) at (0, 0, 0) in component "03_Front_Spinner"
component "Spinner_Motor" placed x (1, 0, 0) y (0, 1, 0) z (0, 0, 1) at (0, 0, 0) in component "03_Front_Spinner"
component "Spinner_Motor_Cradle" placed x (1, 0, 0) y (0, 1, 0) z (0, 0, 1) at (0, 0, 0) in component "03_Front_Spinner"
component "Weapon_Pulley" placed x (1, 0, 0) y (0, 1, 0) z (0, 0, 1) at (0, 0, 0) in component "03_Front_Spinner"
component "Motor_Pulley" placed x (1, 0, 0) y (0, 1, 0) z (0, 0, 1) at (0, 0, 0) in component "03_Front_Spinner"
component "ESC_Tekko32" placed x (1, 0, 0) y (0, 1, 0) z (0, 0, 1) at (0, 0, 0) in component "03_Front_Spinner"
component "Spinner_Bar" placed x (1, 0, 0) y (0, 1, 0) z (0, 0, 1) at (0, 0, 0) in component "03_Front_Spinner"
component "Spinner_Sweep_Envelope" placed x (1, 0, 0) y (0, 1, 0) z (0, 0, 1) at (0, 0, 0) in component "03_Front_Spinner"
component "Cable_Routing_Keepouts" placed x (1, 0, 0) y (0, 1, 0) z (0, 0, 1) at (0, 0, 0) in component "05_Electronics"
component "Battery_and_Tray" placed x (1, 0, 0) y (0, 1, 0) z (0, 0, 1) at (0, 0, 0) in component "05_Electronics"
component "Rx_ER6" placed x (1, 0, 0) y (0, 1, 0) z (0, 0, 1) at (0, 0, 0) in component "05_Electronics"
component "UBEC_5A" placed x (1, 0, 0) y (0, 1, 0) z (0, 0, 1) at (0, 0, 0) in component "05_Electronics"
component "DRV8874_A" placed x (1, 0, 0) y (0, 1, 0) z (0, 0, 1) at (0, 0, 0) in component "05_Electronics"
component "DRV8874_B" placed x (1, 0, 0) y (0, 1, 0) z (0, 0, 1) at (0, 0, 0) in component "05_Electronics"
component "ESP32_DevKit" placed x (1, 0, 0) y (0, 1, 0) z (0, 0, 1) at (0, 0, 0) in component "05_Electronics"
component "FingerTech_Mini_Switch_Envelope" placed x (1, 0, 0) y (0, 1, 0) z (0, 0, 1) at (0, 0, 0) in component "05_Electronics"
component "BBB_Dual_Brushed_ESC_v2_Envelope" placed x (1, 0, 0) y (0, 1, 0) z (0, 0, 1) at (0, 0, 0) in component "05_Electronics"
component "Wire_Clips" placed x (1, 0, 0) y (0, 1, 0) z (0, 0, 1) at (0, 0, 0) in component "06_3D_Printed"
component "Non_Structural_Covers" placed x (1, 0, 0) y (0, 1, 0) z (0, 0, 1) at (0, 0, 0) in component "06_3D_Printed"
component "TPU_Bumpers" placed x (1, 0, 0) y (0, 1, 0) z (0, 0, 1) at (0, 0, 0) in component "06_3D_Printed"
component "Battery_Holder" placed x (1, 0, 0) y (0, 1, 0) z (0, 0, 1) at (0, 0, 0) in component "06_3D_Printed"
component "Batt_Post_1" placed x (1, 0, 0) y (0, 1, 0) z (0, 0, 1) at (0, 0, 0) in component "06_3D_Printed"
component "Batt_Post_2" placed x (1, 0, 0) y (0, 1, 0) z (0, 0, 1) at (0, 0, 0) in component "06_3D_Printed"
component "Batt_Post_3" placed x (1, 0, 0) y (0, 1, 0) z (0, 0, 1) at (0, 0, 0) in component "06_3D_Printed"
component "Batt_Post_4" placed x (1, 0, 0) y (0, 1, 0) z (0, 0, 1) at (0, 0, 0) in component "06_3D_Printed"
component "Disconnect_Post_1" placed x (1, 0, 0) y (0, 1, 0) z (0, 0, 1) at (0, 0, 0) in component "06_3D_Printed"
component "Disconnect_Post_2" placed x (1, 0, 0) y (0, 1, 0) z (0, 0, 1) at (0, 0, 0) in component "06_3D_Printed"
component "Holder_ESC_Tekko32" placed x (1, 0, 0) y (0, 1, 0) z (0, 0, 1) at (0, 0, 0) in component "06_3D_Printed"
component "Holder_Rx_ER6" placed x (1, 0, 0) y (0, 1, 0) z (0, 0, 1) at (0, 0, 0) in component "06_3D_Printed"
component "Holder_UBEC_5A" placed x (1, 0, 0) y (0, 1, 0) z (0, 0, 1) at (0, 0, 0) in component "06_3D_Printed"
component "Holder_DRV8874_A" placed x (1, 0, 0) y (0, 1, 0) z (0, 0, 1) at (0, 0, 0) in component "06_3D_Printed"
component "Holder_DRV8874_B" placed x (1, 0, 0) y (0, 1, 0) z (0, 0, 1) at (0, 0, 0) in component "06_3D_Printed"
component "Holder_ESP32" placed x (1, 0, 0) y (0, 1, 0) z (0, 0, 1) at (0, 0, 0) in component "06_3D_Printed"
component "FingerTech_Switch_Adapter" placed x (1, 0, 0) y (0, 1, 0) z (0, 0, 1) at (0, 0, 0) in component "06_3D_Printed"
component "Rear_Panel" placed x (1, 0, 0) y (0, 1, 0) z (0, 0, 1) at (0, 0, 0) in component "Non_Structural_Covers"
component "06_3D_Printed" placed x (1, 0, 0) y (0, 1, 0) z (0, 0, 1) at (0, 0, 0) in component "TPU_Bumpers"
component "Lifter_Spatula_62mm" placed x (1, 0, 0) y (0, 1, 0) z (0, 0, 1) at (0, 0, 0) in component "07_Wedge_Lifter_Option"
component "Lifter_Hinge_Boss" placed x (1, 0, 0) y (0, 1, 0) z (0, 0, 1) at (0, 0, 0) in component "07_Wedge_Lifter_Option"
component "Lifter_Pivot_Support_L" placed x (1, 0, 0) y (0, 1, 0) z (0, 0, 1) at (0, 0, 0) in component "07_Wedge_Lifter_Option"
component "Lifter_Pivot_Support_R" placed x (1, 0, 0) y (0, 1, 0) z (0, 0, 1) at (0, 0, 0) in component "07_Wedge_Lifter_Option"
component "Lifter_Pivot_Pin_6mm" placed x (1, 0, 0) y (0, 1, 0) z (0, 0, 1) at (0, 0, 0) in component "07_Wedge_Lifter_Option"
component "Servo_30kgcm_Envelope_Only" placed x (1, 0, 0) y (0, 1, 0) z (0, 0, 1) at (0, 0, 0) in component "07_Wedge_Lifter_Option"
component "Lifter_Servo_Horn_Envelope_Only" placed x (1, 0, 0) y (0, 1, 0) z (0, 0, 1) at (0, 0, 0) in component "07_Wedge_Lifter_Option"
component "Lifter_Linkage_Envelope_Only" placed x (1, 0, 0) y (0, 1, 0) z (0, 0, 1) at (0, 0, 0) in component "07_Wedge_Lifter_Option"
component "Repeat_40kg_Servo_MaxEnvelope" placed x (1, 0, 0) y (0, 1, 0) z (0, 0, 1) at (0, 0, 0) in component "07_Wedge_Lifter_Option"
component "Lifter_Servo_Base_Rail_L" placed x (1, 0, 0) y (0, 1, 0) z (0, 0, 1) at (0, 0, 0) in component "07_Wedge_Lifter_Option"
component "Lifter_Servo_Base_Rail_R" placed x (1, 0, 0) y (0, 1, 0) z (0, 0, 1) at (0, 0, 0) in component "07_Wedge_Lifter_Option"
component "Lifter_Aluminium_Horn" placed x (1, 0, 0) y (0, 1, 0) z (0, 0, 1) at (0, 0, 0) in component "07_Wedge_Lifter_Option"
component "Lifter_Connecting_Rod" placed x (1, 0, 0) y (0, 1, 0) z (0, 0, 1) at (0, 0, 0) in component "07_Wedge_Lifter_Option"
component "Lifter_Lower_Hard_Stop" placed x (1, 0, 0) y (0, 1, 0) z (0, 0, 1) at (0, 0, 0) in component "07_Wedge_Lifter_Option"
component "Lifter_Servo_Clamp_Bar_L" placed x (1, 0, 0) y (0, 1, 0) z (0, 0, 1) at (0, 0, 0) in component "07_Wedge_Lifter_Option"
component "Lifter_Servo_Clamp_Post_L_Rear" placed x (1, 0, 0) y (0, 1, 0) z (0, 0, 1) at (0, 0, 0) in component "07_Wedge_Lifter_Option"
component "Lifter_Servo_Clamp_Post_L_Front" placed x (1, 0, 0) y (0, 1, 0) z (0, 0, 1) at (0, 0, 0) in component "07_Wedge_Lifter_Option"
component "Lifter_Servo_Clamp_Bar_R" placed x (1, 0, 0) y (0, 1, 0) z (0, 0, 1) at (0, 0, 0) in component "07_Wedge_Lifter_Option"
component "Lifter_Servo_Clamp_Post_R_Rear" placed x (1, 0, 0) y (0, 1, 0) z (0, 0, 1) at (0, 0, 0) in component "07_Wedge_Lifter_Option"
component "Lifter_Servo_Clamp_Post_R_Front" placed x (1, 0, 0) y (0, 1, 0) z (0, 0, 1) at (0, 0, 0) in component "07_Wedge_Lifter_Option"
component "Lifter_Pin_C_Clip_L" placed x (1, 0, 0) y (0, 1, 0) z (0, 0, 1) at (0, 0, 0) in component "07_Wedge_Lifter_Option"
component "Lifter_Pin_C_Clip_R" placed x (1, 0, 0) y (0, 1, 0) z (0, 0, 1) at (0, 0, 0) in component "07_Wedge_Lifter_Option"
component "Grabber_Upper_Jaw" placed x (1, 0, 0) y (0, 1, 0) z (0, 0, 1) at (0, 0, 0) in component "08_Grabber_Addon_Option"
component "Grabber_Arm_L" placed x (1, 0, 0) y (0, 1, 0) z (0, 0, 1) at (0, 0, 0) in component "08_Grabber_Addon_Option"
component "Grabber_Arm_R" placed x (1, 0, 0) y (0, 1, 0) z (0, 0, 1) at (0, 0, 0) in component "08_Grabber_Addon_Option"
component "Grabber_Pivot_Pin_6mm" placed x (1, 0, 0) y (0, 1, 0) z (0, 0, 1) at (0, 0, 0) in component "08_Grabber_Addon_Option"
component "Grabber_Pivot_Bracket_L" placed x (1, 0, 0) y (0, 1, 0) z (0, 0, 1) at (0, 0, 0) in component "08_Grabber_Addon_Option"
component "Grabber_Pivot_Bracket_R" placed x (1, 0, 0) y (0, 1, 0) z (0, 0, 1) at (0, 0, 0) in component "08_Grabber_Addon_Option"
component "Grabber_Second_Servo_Envelope_Only" placed x (1, 0, 0) y (0, 1, 0) z (0, 0, 1) at (0, 0, 0) in component "08_Grabber_Addon_Option"
component "Grabber_Linkage_Envelope_Only" placed x (1, 0, 0) y (0, 1, 0) z (0, 0, 1) at (0, 0, 0) in component "08_Grabber_Addon_Option"
component "BBB_22mm_Gearmotor_L" placed x (1, 0, 0) y (0, 1, 0) z (0, 0, 1) at (0, 0, 0) in component "09_3S_Drive_Upgrade"
component "BBB_4mm_Output_Shaft_L" placed x (1, 0, 0) y (0, 1, 0) z (0, 0, 1) at (0, 0, 0) in component "09_3S_Drive_Upgrade"
component "BBB_Face_Mount_26mm_L" placed x (1, 0, 0) y (0, 1, 0) z (0, 0, 1) at (0, 0, 0) in component "09_3S_Drive_Upgrade"
component "BBB_Motor_Cradle_L" placed x (1, 0, 0) y (0, 1, 0) z (0, 0, 1) at (0, 0, 0) in component "09_3S_Drive_Upgrade"
component "Repeat_4mm_Clamp_Hub_L" placed x (1, 0, 0) y (0, 1, 0) z (0, 0, 1) at (0, 0, 0) in component "09_3S_Drive_Upgrade"
component "BBB_22mm_Gearmotor_R" placed x (1, 0, 0) y (0, 1, 0) z (0, 0, 1) at (0, 0, 0) in component "09_3S_Drive_Upgrade"
component "BBB_4mm_Output_Shaft_R" placed x (1, 0, 0) y (0, 1, 0) z (0, 0, 1) at (0, 0, 0) in component "09_3S_Drive_Upgrade"
component "BBB_Face_Mount_26mm_R" placed x (1, 0, 0) y (0, 1, 0) z (0, 0, 1) at (0, 0, 0) in component "09_3S_Drive_Upgrade"
component "BBB_Motor_Cradle_R" placed x (1, 0, 0) y (0, 1, 0) z (0, 0, 1) at (0, 0, 0) in component "09_3S_Drive_Upgrade"
component "Repeat_4mm_Clamp_Hub_R" placed x (1, 0, 0) y (0, 1, 0) z (0, 0, 1) at (0, 0, 0) in component "09_3S_Drive_Upgrade"
component "Battery_Clamp_Bar_1" placed x (1, 0, 0) y (0, 1, 0) z (0, 0, 1) at (0, 0, 0) in component "10_Battery_Restraints"
component "Battery_Clamp_Bar_2" placed x (1, 0, 0) y (0, 1, 0) z (0, 0, 1) at (0, 0, 0) in component "10_Battery_Restraints"
equation "body_L = 180 mm" comment "Body length"
equation "body_W = 160 mm" comment "Body width incl. wheels"
equation "body_H = 80 mm" comment "Chassis height - raised from 70mm to give spinner sweep safe clearance under top cover"
equation "base_t = 2 mm" comment "DECIDED 2026-09-23: 2 mm aluminium plate (user approved)"
equation "side_t = 2 mm" comment "DECIDED 2026-09-23: 2 mm aluminium plate (user approved)"
equation "ground_clearance = 3 mm" comment "Ground clearance target"
equation "wheel_OD = 42 mm" comment "CONFIRMED: 42mm TT-motor wheel"
equation "wheel_W = 19 mm" comment "CONFIRMED (typical TT wheel width; verify against actual supplier spec)"
equation "motor_OD = 25 mm" comment "Gear motor housing envelope"
equation "pcb_L = 60 mm" comment "Control PCB placeholder length"
equation "pcb_W = 50 mm" comment "Control PCB placeholder width"
equation "pcb_keepout_H = 22 mm" comment "PCB top keepout height (placeholder)"
equation "assembly_clearance = 1 mm" comment "Generic assembly clearance"
equation "d14 = body_W"
equation "d15 = body_L"
equation "d16 = wheel_W"
equation "d17 = wheel_OD"
equation "d18 = wheel_W"
equation "d19 = wheel_OD"
equation "d20 = pcb_W"
equation "d21 = pcb_L"
equation "d26 = body_W"
equation "d27 = body_L"
equation "d28 = -base_t"
equation "d56 = -body_W / 2"
equation "d58 = body_H - base_t"
equation "d59 = body_L"
equation "d60 = side_t"
equation "d62 = body_W / 2"
equation "d64 = body_H - base_t"
equation "d65 = body_L"
equation "d66 = -side_t"
equation "d68 = -body_W / 2"
equation "d70 = wheel_OD"
equation "d71 = wheel_W"
equation "d73 = body_W / 2"
equation "d75 = wheel_OD"
equation "d76 = -wheel_W"
equation "spinner_gap_W = 70 mm" comment "MOCK layout gap for front spinner - NOT_FOR_MANUFACTURING, confirm with real weapon assembly"
equation "wedge_depth = 50 mm" comment "MOCK front wedge depth (front-to-back) - NOT_FOR_MANUFACTURING placeholder"
equation "d104 = body_H - base_t"
equation "d106 = body_W"
equation "d107 = body_L"
equation "d108 = base_t"
equation "battery_mock_L = 104 mm" comment "CONFIRMED: 3S 2200mAh LiPo typical size (Turnigy/GNB-class, ~500-700 THB Thai retail)"
equation "battery_mock_W = 35 mm" comment "MOCK 3S LiPo envelope width - NOT_FOR_MANUFACTURING"
equation "battery_mock_H = 27 mm" comment "MOCK 3S LiPo envelope height - NOT_FOR_MANUFACTURING"
equation "pcb_t = 1.6 mm" comment "Standard PCB thickness placeholder"
equation "module_mock_L = 25 mm" comment "MOCK small electronics module envelope length (driver/BEC/receiver/disconnect) - NOT_FOR_MANUFACTURING"
equation "module_mock_W = 20 mm" comment "MOCK small electronics module envelope width - NOT_FOR_MANUFACTURING"
equation "module_mock_H = 10 mm" comment "MOCK small electronics module envelope height - NOT_FOR_MANUFACTURING"
equation "tt_gearbox_L = 24 mm" comment "TT motor gearbox length along shaft axis - TYPICAL VALUE, confirm exact supplier datasheet before drilling mount holes"
equation "tt_gearbox_W = 22 mm" comment "TT motor gearbox cross-section width - TYPICAL VALUE, confirm before mount holes"
equation "tt_gearbox_H = 18 mm" comment "TT motor gearbox cross-section height - TYPICAL VALUE, confirm before mount holes"
equation "tt_can_D = 20 mm" comment "TT motor can (motor body) diameter - TYPICAL VALUE"
equation "tt_can_L = 25 mm" comment "TT motor can (motor body) length - TYPICAL VALUE"
equation "tt_shaft_D = 5 mm" comment "TT motor output D-shaft diameter - TYPICAL VALUE, confirm before hub fit"
equation "tt_shaft_L = 10 mm" comment "TT motor output shaft protrusion length - TYPICAL VALUE"
equation "d208 = wheel_OD / 2"
equation "d209 = wheel_OD / 2"
equation "d218 = side_t * 5"
equation "d220 = side_t * 5"
equation "d222 = side_t * 5"
equation "d224 = side_t * 5"
equation "d226 = -body_W / 2 + wheel_W"
equation "d228 = tt_gearbox_H"
equation "d229 = tt_gearbox_W"
equation "d230 = tt_gearbox_L"
equation "d234 = tt_can_D"
equation "d237 = -tt_can_L"
equation "d239 = body_W / 2 - wheel_W"
equation "d241 = tt_gearbox_H"
equation "d242 = tt_gearbox_W"
equation "d243 = -tt_gearbox_L"
equation "d247 = tt_can_D"
equation "d250 = tt_can_L"
equation "hammer_servo_L = 40.5 mm" comment "CONFIRMED: DS3218MG servo body length (incl. mount tabs), srituhobby.com listing"
equation "hammer_servo_W = 20 mm" comment "CONFIRMED: DS3218MG servo body width"
equation "hammer_servo_H = 40.5 mm" comment "CONFIRMED: DS3218MG servo body height"
equation "hammer_servo_horn_D = 25 mm" comment "MOCK: typical servo horn/spline envelope diameter"
equation "hammer_arm_L = 80 mm" comment "MOCK hammer arm length from pivot to head - NOT_FOR_MANUFACTURING, confirm reach vs chassis geometry"
equation "hammer_head_L = 30 mm" comment "MOCK hammer head length - NOT_FOR_MANUFACTURING"
equation "hammer_head_W = 20 mm" comment "MOCK hammer head width - NOT_FOR_MANUFACTURING"
equation "hammer_head_H = 15 mm" comment "MOCK hammer head height - NOT_FOR_MANUFACTURING"
equation "spinner_motor_D = 27.5 mm" comment "CONFIRMED: A2212 brushless motor can diameter (standard size)"
equation "spinner_motor_L = 30 mm" comment "CONFIRMED: A2212 brushless motor can length (standard size)"
equation "spinner_shaft_D = 4 mm" comment "DECIDED 2026-09-23: 4 mm weapon shaft (separate from the A2212 3.17 mm motor shaft; driven by 1:1 belt) to fit the 624 bearing"
equation "spinner_bearing_OD = 13 mm" comment "DECIDED 2026-09-23: 624 bearing, 4x13x5 mm, bore matches spinner_shaft_D"
equation "spinner_bar_L = 65 mm" comment "MOCK spinner weapon bar length (within spinner_gap_W envelope) - NOT_FOR_MANUFACTURING, needs structural review before fabrication"
equation "spinner_bar_W = 20 mm" comment "MOCK spinner weapon bar width - NOT_FOR_MANUFACTURING"
equation "spinner_bar_T = 6 mm" comment "MOCK spinner weapon bar thickness - NOT_FOR_MANUFACTURING"
equation "esc_L = 45 mm" comment "MOCK typical 30A BLHeli ESC envelope length"
equation "esc_W = 26 mm" comment "MOCK typical 30A ESC envelope width"
equation "esc_H = 8 mm" comment "MOCK typical 30A ESC envelope height"
equation "print_wall_t = 2 mm" comment "3D printed wall thickness placeholder (PETG typical)"
equation "d430 = battery_mock_L"
equation "d431 = battery_mock_W"
equation "d432 = battery_mock_H"
equation "d464 = base_t * 5"
equation "d466 = base_t * 5"
equation "d470 = ground_clearance + base_t"
equation "d473 = ground_clearance + base_t"
equation "d476 = ground_clearance + base_t"
equation "d485 = ground_clearance + base_t"
equation "d486 = -body_W / 2"
equation "d488 = wedge_depth"
equation "d489 = body_H - base_t"
equation "d490 = body_L / 2"
equation "d491 = ( body_W - spinner_gap_W ) / 2"
equation "d495 = ground_clearance + base_t"
equation "d496 = body_W / 2"
equation "d498 = wedge_depth"
equation "d499 = body_H - base_t"
equation "d500 = body_L / 2"
equation "d501 = -( body_W - spinner_gap_W ) / 2"
equation "d505 = ground_clearance + base_t"
equation "d508 = spinner_shaft_D"
equation "d513 = spinner_bearing_OD"
equation "d518 = spinner_bearing_OD"
equation "d528 = spinner_motor_D"
equation "m3_clear_d = 3.4 mm" comment "M3 clearance hole dia for CNC/laser-cut aluminum (tight fit)"
equation "m3_clear_d_fdm = 3.6 mm" comment "M3 clearance hole dia for FDM-printed parts (extra 0.2mm for print tolerance)"
equation "standoff_od = 6 mm" comment "M3 corner standoff outer diameter"
equation "standoff_bore_d = 3.2 mm" comment "Standoff through-bore for M3 screw (tap or use nut at one end)"
equation "tt_hole_spacing = 17.5 mm" comment "CONFIRMED: TT motor (all-metal gearbox variant) 2-hole M3 mount spacing, handsontec.com FAM1062 datasheet - verify against exact purchased unit"
equation "a2212_hole_x = 16 mm" comment "CONFIRMED: A2212 brushless motor rear mount hole spacing (short side), widely documented standard"
equation "a2212_hole_y = 19 mm" comment "CONFIRMED: A2212 brushless motor rear mount hole spacing (long side)"
equation "servo_flange_spacing = 49.5 mm" comment "CONFIRMED: standard servo flange mounting hole spacing (DS3218/MG996R-class), servodatabase.com"
equation "mount_plate_t = 3 mm" comment "Motor mounting bracket/plate thickness (aluminum)"
equation "d563 = standoff_od"
equation "d564 = standoff_bore_d"
equation "d565 = standoff_od"
equation "d566 = standoff_bore_d"
equation "d567 = standoff_od"
equation "d568 = standoff_bore_d"
equation "d569 = standoff_od"
equation "d570 = standoff_bore_d"
equation "d578 = side_t * 5"
equation "d580 = side_t * 5"
equation "d582 = tt_gearbox_L * 3"
equation "d584 = tt_gearbox_L * 3"
equation "d586 = spinner_motor_L * 3"
equation "d588 = base_t * 4"
equation "lip_h = 5 mm" comment "Battery holder side-lip height"
equation "strap_slot_w = 10 mm" comment "Battery strap slot width"
equation "strap_slot_l = 4 mm" comment "Battery strap slot length (thin slit)"
equation "pcb_standoff_h = 3 mm" comment "PCB standoff height (raises board off floor)"
equation "m2_5_clear_d_fdm = 2.9 mm" comment "M2.5 clearance hole for FDM-printed standoffs"
equation "d597 = battery_mock_L"
equation "d598 = battery_mock_W"
equation "d599 = print_wall_t"
equation "d601 = print_wall_t * 5"
equation "d605 = lip_h"
equation "d607 = lip_h"
equation "d639 = base_t * 6"
equation "d641 = base_t * 6"
equation "d643 = base_t * 6"
equation "d645 = base_t * 6"
equation "d657 = side_t * 6"
equation "d659 = side_t * 6"
equation "m2_clear_d = 2.2 mm" comment "M2 clearance hole for small electronics module mounting"
equation "roll_pin_d = 2 mm" comment "Roll pin diameter through shaft+bar - shock-resistant weapon fastening, stronger than friction set-screw alone"